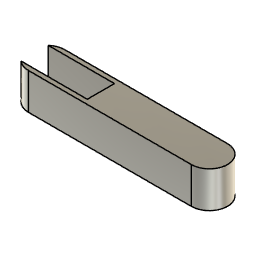
Finger v1 (Autodesk Fusion 360 design; units mm, degrees)
Autodesk Fusion 360 part; units mm, degrees
sketch "Sketch1" plane through (0, 0, 0) normal (0, 0, 1) x (1, 0, 0)
  line L0 (0, 0) -> (45, 0)
  line L1 (45, 10) -> (0, 10)
  arc A0 (0, 10) -> (0, 0) centre (0, 5) ccw
  arc A1 (45, 0) -> (45, 10) centre (45, 5) ccw
  dimension "d1" = 10
  dimension "d2" = 45
  constraint horizontal L0
  constraint horizontal L1
  constraint coincident L0.start A0.end
  constraint tangent L1 A0
  constraint coincident L0.start A0
  constraint tangent L0 A1
  constraint coincident L0 A0.end
  constraint tangent L1 A1
  constraint tangent L0 A0
  measures "d1" distance of L0.start L1.end
  measures "d2" distance of A0.centre A1.centre
extrude "Extrude1" add sketch "Sketch1" along normal blind 10
sketch "Sketch2" plane through (0, 0, 0) normal (1, 0, 0) x (0, 1, 0)
  line L0 (1.25, 1.25) -> (8.75, 1.25)
  line L1 (8.75, 1.25) -> (8.75, 8.75)
  line L2 (8.75, 8.75) -> (1.25, 8.75)
  line L3 (1.25, 8.75) -> (1.25, 1.25)
  line L4 (10, 1.25) -> (8.75, 1.25) construction
  line L5 (0, 1.25) -> (1.25, 1.25) construction
  line L6 (0, 0) -> (0, 10)
  line L7 (10, 0) -> (10, 10)
  line L8 (8.75, 8.75) -> (8.75, 10) construction
  line L9 (8.75, 1.25) -> (8.75, 0) construction
  line L10 (10, 0) -> (0, 0)
  line L11 (10, 10) -> (0, 10)
  point P0 (10, 0)
  dimension "d5" = 7.5
  dimension "d6" = 7.5
  constraint horizontal L0
  constraint vertical L1
  constraint horizontal L2
  constraint vertical L3
  constraint perpendicular L1 L4
  constraint parallel L0 L5
  constraint coincident L0.start L3.end
  constraint coincident L0.end L1.start
  constraint equal L4 L5
  constraint coincident L5.start L6
  constraint coincident L4.start L7
  constraint perpendicular L2 L8
  constraint perpendicular L0 L9
  constraint coincident L9.end L10
  constraint coincident L8.end L11
  constraint equal L8 L9
  measures "d5" distance of L0.start L0.end
  measures "d6" distance of L0.start L2.end
extrude "Extrude2" cut sketch "Sketch2" along normal blind 45 and the other way through all contours L0 L1 L2 L3
sketch "Sketch3" plane through (0, 0, 10) normal (0, 0, 1) x (-1, 0, 0)
  arc A0 (-45, 0) -> (-45, -10) centre (-45, -5) ccw
  line L0 (-45, -10) -> (0, -10)
  arc A1 (0, -10) -> (0, 0) centre (0, -5) ccw
  line L1 (0, 0) -> (-45, 0)
  line L2 (5, -8.75) -> (-15, -8.75)
  line L3 (-15, -8.75) -> (-15, -1.25)
  line L4 (-15, -1.25) -> (5, -1.25)
  line L5 (5, -1.25) -> (5, -8.75)
  line L6 (5, -8.75) -> (5, -10) construction
  line L7 (5, -1.25) -> (5, 0) construction
  dimension "d11" = 7.5
  dimension "d12" = 30
  constraint horizontal L2
  constraint vertical L3
  constraint horizontal L4
  constraint vertical L5
  constraint tangent A1 L5
  constraint vertical L6
  constraint perpendicular L4 L7
  constraint coincident L2.start L5.end
  constraint equal L6 L7
  constraint horizontal L0.end L6.end
  constraint horizontal A1.end L7.end
  measures "d11" distance of L2.start L4.end
  measures "d12" distance of A0.centre L3
extrude "Extrude3" cut sketch "Sketch3" against normal up to surface (1.25 mm away) contours A1 L2 L3 L4
